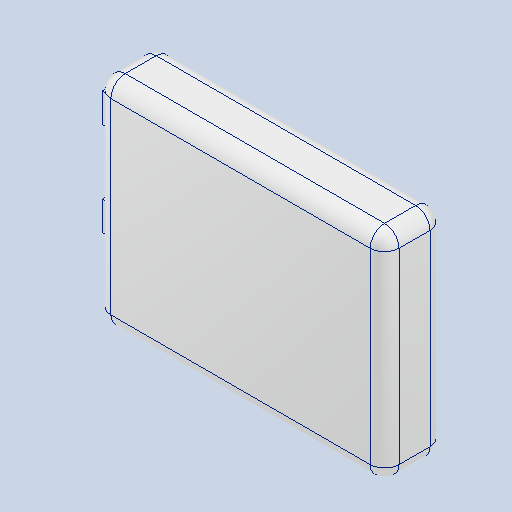
# Autodesk Inventor part: 803048
Saved by Autodesk Inventor 2022 (Build 260153000, 153)
## iProperties
Created: 2022-01-07
Part Number: 803048
Material: Алюминий 6061
Document SubType Name: Modeling
Designer: Me
Density: 2.7 g/cm^3
Appearance: Алюминий — плоский
Author: Me
Autodesk Inventor part; units mm, degrees
ref_plane "YZ Plane" through (0, 0, 0) normal (1, 0, 0) x (0, 1, 0)
ref_plane "XZ Plane" through (0, 0, 0) normal (0, 1, 0) x (-1, 0, 0)
ref_plane "XY Plane" through (0, 0, 0) normal (0, 0, 1) x (1, 0, 0)
sketch "Эскиз1" plane through (0, 0, 0) normal (0, 0, 1) x (1, 0, 0)
  line L0 (-13.4163, 13.7539) -> (26.5837, 13.7539)
  line L1 (26.5837, 13.7539) -> (26.5837, -16.2461)
  line L2 (26.5837, -16.2461) -> (-13.4163, -16.2461)
  line L3 (-13.4163, -16.2461) -> (-13.4163, 13.7539)
  point P0 (0, 0)
  dimension "d0" = 40
  dimension "d1" = 30
  constraints: 8 end point, 2 parallel, 1 horizontal, 1 perpendicular
  measures "d0" distance of L0.start L0.end
  measures "d1" distance of L0.end L1.end
extrude "Выдавливание1" add sketch "Эскиз1" along normal blind 8.3
sketch "Эскиз2" plane through (-13.4163, -16.2461, 0) normal (-1, 0, 0) x (0, 0, 1)
  line L0 (3, 6.5) -> (3.5, 6.5)
  line L1 (3.5, 6.5) -> (3.5, 10.5)
  line L2 (3.5, 10.5) -> (3, 10.5)
  line L3 (3, 10.5) -> (3, 6.5)
  line L4 (3, 19.5) -> (3.5, 19.5)
  line L5 (3.5, 19.5) -> (3.5, 23.5)
  line L6 (3.5, 23.5) -> (3, 23.5)
  line L7 (3, 23.5) -> (3, 19.5)
  line L8 (0, 0) -> (8.3, 0) projected
  line L9 (0, 30) -> (0, 0) projected
  point P0 (0, 16.2461)
  dimension "d4" = 4
  dimension "d5" = 4
  dimension "d6" = 0.5
  dimension "d7" = 0.5
  dimension "d8" = 9
  dimension "d9" = 6.5
  dimension "d10" = 3
  constraints: 16 end point, 4 parallel, 2 horizontal, 2 perpendicular, 2 point on line
  measures "d4" distance of L2.end L0.start
  measures "d5" distance of L6.end L4.start
  measures "d6" distance of L0.start L0.end
  measures "d7" distance of L4.start L4.end
  measures "d8" distance between parallel lines of L2 L4
  measures "d9" distance between parallel lines of L8 L0
  measures "d10" distance between parallel lines of L9 L3
extrude "Выдавливание2" add sketch "Эскиз2" along normal blind 4
fillet "Сопряжение1" radius 2 12 edges at (6.5837, 13.7539, 8.3) (6.5837, 13.7539, 0) (6.5837, -16.2461, 8.3) (6.5837, -16.2461, 0) (26.5837, -1.2461, 0) (26.5837, -1.2461, 8.3) (26.5837, -16.2461, 4.15) (-13.4163, -1.2461, 0) (-13.4163, -16.2461, 4.15) (-13.4163, 13.7539, 4.15) (-13.4163, -1.2461, 8.3) (26.5837, 13.7539, 4.15)
